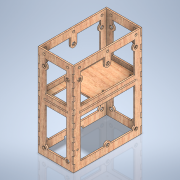
# Autodesk Inventor part: Skeleton
Saved by Autodesk Inventor 2020.2 (Build 242310000, 310)
## iProperties
Created: 2020-03-04
Part Number: Skeleton
Material: Wood (Birch)
Document SubType Name: Modeling
Designer: sdekr
Density: 0.55 g/cm^3
Appearance: Birch - Natural Polished
Author: sdekr
Autodesk Inventor part; units mm, degrees
sketch "Sketch1" plane through (0, 0, 0) normal (0, 1, 0) x (-1, 0, 0)
  line L0 (-37.5, 72.5) -> (37.5, 72.5)
  line L1 (37.5, 72.5) -> (37.5, -72.5)
  line L2 (37.5, -72.5) -> (-37.5, -72.5)
  line L3 (-37.5, -72.5) -> (-37.5, 72.5)
  line L4 (-37.5, 72.5) -> (37.5, -72.5) construction
  line L5 (37.5, 72.5) -> (-37.5, -72.5) construction
  point P0 (0, 0)
  dimension "d0" = 75
  dimension "d1" = 145
  constraints: 12 end point, 2 midpoint, 2 parallel, 1 horizontal, 1 perpendicular
  measures "d0" distance of L1.end L2.end
  measures "d1" distance of L0.end L1.end
surface extrude "ExtrusionSrf1" sketch "Sketch1" along normal blind 195 shown yes curves L0 L1 L2 L3
sketch "Sketch2" plane through (-37.5, 0, 72.5) normal (0, 0, 1) x (1, 0, 0)
  line L0 (0, 195) -> (75, 195) projected
  line L1 (75, 0) -> (75, 195) projected
  line L2 (0, 195) -> (75, 195)
  line L3 (75, 195) -> (75, 0)
  line L4 (75, 0) -> (0, 0)
  line L5 (0, 0) -> (0, 195)
  line L6 (15, 180) -> (60, 180)
  line L7 (60, 180) -> (60, 115)
  line L8 (60, 115) -> (15, 115)
  line L9 (15, 115) -> (15, 180)
  line L10 (15, 95) -> (60, 95)
  line L11 (60, 95) -> (60, 15)
  line L12 (60, 15) -> (15, 15)
  line L13 (15, 15) -> (15, 95)
  circle A0 centre (12.5, 187.5) radius 2.4
  circle A1 centre (62.5, 187.5) radius 2.4
  point P0 (37.5, 0)
  dimension "d4" = 15
  dimension "d5" = 15
  dimension "d6" = 15
  dimension "d7" = 15
  dimension "d8" = 15
  dimension "d9" = 20
  dimension "d12" = 4.8
  dimension "d13" = 4.8
  dimension "d14" = 7.5
  dimension "d15" = 7.5
  dimension "d16" = 12.5
  dimension "d17" = 12.5
  dimension "d81" = 80
  constraints: 24 end point, 6 parallel, 3 horizontal, 3 perpendicular, 2 centre point, 1 point on line
  measures "d4" distance between parallel lines of L1 L7
  measures "d5" distance between parallel lines of L5 L9
  measures "d6" distance between parallel lines of L4 L12
  measures "d7" distance between parallel lines of L0 L6
  measures "d8" distance between parallel lines of L5 L13
  measures "d9" distance between parallel lines of L10 L8
  measures "d12" diameter of A0
  measures "d13" diameter of A1
  measures "d14" distance from line of L0 A1.centre
  measures "d15" distance from line of L0 A0.centre
  measures "d16" distance from line of L5 A0.centre
  measures "d17" distance from line of L1 A1.centre
  measures "d81" distance of L10.end L11.end
extrude "Extrusion1" add sketch "Sketch2" against normal blind 3
ref_plane "Work Plane1" through (-37.5, 0, 0) normal (0, 0, 1) x (1, 0, 0)
sketch "Sketch5" plane through (-37.5, 0, 72.5) normal (0, 0, 1) x (1, 0, 0)
  line L0 (75, 0) -> (75, 195) projected
  line L1 (75, 180) -> (72, 180)
  line L2 (72, 180) -> (72, 165)
  line L3 (72, 165) -> (75, 165)
  line L4 (75, 165) -> (75, 180)
  line L5 (75, 195) -> (0, 195) projected
  line L6 (75, 155) -> (72, 155)
  line L7 (72, 155) -> (72, 140)
  line L8 (72, 140) -> (75, 140)
  line L9 (75, 140) -> (75, 155)
  line L10 (75, 130) -> (72, 130)
  line L11 (72, 130) -> (72, 115)
  line L12 (72, 115) -> (75, 115)
  line L13 (75, 115) -> (75, 130)
  line L14 (75, 105) -> (72, 105)
  line L15 (72, 105) -> (72, 90)
  line L16 (72, 90) -> (75, 90)
  line L17 (75, 90) -> (75, 105)
  line L18 (75, 80) -> (72, 80)
  line L19 (72, 80) -> (72, 65)
  line L20 (72, 65) -> (75, 65)
  line L21 (75, 65) -> (75, 80)
  line L22 (0, 0) -> (75, 0) projected
  line L23 (62.5, 106.5) -> (12.5, 106.5)
  line L24 (12.5, 106.5) -> (12.5, 103.5)
  line L25 (12.5, 103.5) -> (62.5, 103.5)
  line L26 (62.5, 103.5) -> (62.5, 106.5)
  line L27 (0, 195) -> (0, 0) projected
  line L28 (75, 55) -> (72, 55)
  line L29 (72, 55) -> (72, 40)
  line L30 (72, 40) -> (75, 40)
  line L31 (75, 40) -> (75, 55)
  line L32 (75, 30) -> (72, 30)
  line L33 (72, 30) -> (72, 15)
  line L34 (72, 15) -> (75, 15)
  line L35 (75, 15) -> (75, 30)
  line L36 (60, 115) -> (15, 115) projected
  line L37 (15, 95) -> (60, 95) projected
  point P0 (37.5, 0)
  point P1 (75, 90)
  point P2 (75, 65)
  point P3 (75, 115)
  point P4 (75, 140)
  point P5 (75, 165)
  point P6 (12.5, 105)
  point P7 (37.5, 103.5)
  point P8 (37.5, 195)
  dimension "d38" = 3
  dimension "d39" = 15
  dimension "d43" = 25
  dimension "d59" = 3
  dimension "d60" = 50
  dimension "d73" = 15
  dimension "d74" = 15
  dimension "d82" = 8.5
  dimension "d125" = 8.5
  constraints: 64 end point, 4 parallel, 3 midpoint, 2 horizontal, 2 perpendicular, 1 point on line, 1 vertical, 1 vertical alignment, 48 other
  measures "d38" distance of L1.start L1.end
  measures "d39" distance of L1.end L2.end
  measures "d43" distance of L1.start L6.start
  measures "d59" distance of L25.end L23.start
  measures "d60" distance of L23.start L23.end
  measures "d73" distance between parallel lines of L5 L1
  measures "d74" distance between parallel lines of L34 L22
  measures "d82" distance between parallel lines of L36 L23
  measures "d125" distance between parallel lines of L37 L25
extrude "Extrusion4" cut sketch "Sketch5" against normal up to surface (3 mm away) contours L34 L33 L32 L0 | L30 L29 L28 L0 | L0 L3 L2 L1 | L20 L19 L18 L0 | L0 L8 L7 L6 | L16 L15 L14 L0 | L0 L12 L11 L10 | L26 L25 L24 L23
ref_plane "Work Plane4" through (0, 195, 72.5) normal (1, 0, 0) x (0, 0, -1)
mirror "Mirror3" about plane through (0, 195, 72.5) normal (1, 0, 0) of "Extrusion4"
sketch "Sketch11" plane through (-37.5, 0, 69.5) normal (0, 0, -1) x (-1, 0, 0)
  circle A0 centre (-12.5, 165) radius 2.4 projected
  circle A1 centre (-62.5, 165) radius 2.4 projected
  circle A2 centre (-12.5, 15) radius 2.4 projected
  circle A3 centre (-62.5, 15) radius 2.4 projected
  line L0 (-60.6236, 168.25) -> (-58.7472, 165)
  line L1 (-58.7472, 165) -> (-60.6236, 161.75)
  line L2 (-60.6236, 161.75) -> (-64.3764, 161.75)
  line L3 (-64.3764, 161.75) -> (-66.2528, 165)
  line L4 (-66.2528, 165) -> (-64.3764, 168.25)
  line L5 (-64.3764, 168.25) -> (-60.6236, 168.25)
  line L6 (-14.3764, 168.25) -> (-10.6236, 168.25)
  line L7 (-10.6236, 168.25) -> (-8.7472, 165)
  line L8 (-8.7472, 165) -> (-10.6236, 161.75)
  line L9 (-10.6236, 161.75) -> (-14.3764, 161.75)
  line L10 (-14.3764, 161.75) -> (-16.2528, 165)
  line L11 (-16.2528, 165) -> (-14.3764, 168.25)
  line L12 (-10.6236, 18.25) -> (-8.7472, 15)
  line L13 (-8.7472, 15) -> (-10.6236, 11.75)
  line L14 (-10.6236, 11.75) -> (-14.3764, 11.75)
  line L15 (-14.3764, 11.75) -> (-16.2528, 15)
  line L16 (-16.2528, 15) -> (-14.3764, 18.25)
  line L17 (-14.3764, 18.25) -> (-10.6236, 18.25)
  line L18 (-60.6236, 18.25) -> (-58.7472, 15)
  line L19 (-58.7472, 15) -> (-60.6236, 11.75)
  line L20 (-60.6236, 11.75) -> (-64.3764, 11.75)
  line L21 (-64.3764, 11.75) -> (-66.2528, 15)
  line L22 (-66.2528, 15) -> (-64.3764, 18.25)
  line L23 (-64.3764, 18.25) -> (-60.6236, 18.25)
  circle A4 centre (-62.5, 165) radius 7
  circle A5 centre (-12.5, 165) radius 7
  circle A6 centre (-12.5, 15) radius 7
  circle A7 centre (-62.5, 15) radius 7
  point P0 (-37.5, 0)
  point P1 (-62.5, 18.25)
  dimension "d89" = 6.5
  dimension "d90" = 6.5
  dimension "d91" = 6.5
  dimension "d92" = 6.5
  dimension "d93" = 14
  dimension "d94" = 14
  dimension "d95" = 14
  dimension "d96" = 14
  constraints: 48 end point, 7 coincident, 4 centre point, 2 horizontal, 1 midpoint, 1 point on line, 52 other
  measures "d89" distance from line of point (-62.5, 18.25) L20
  measures "d90" distance between parallel lines of L14 L17
  measures "d91" distance between parallel lines of L2 L5
  measures "d92" distance between parallel lines of L9 L6
  measures "d93" diameter of A4
  measures "d94" diameter of A5
  measures "d95" diameter of A6
  measures "d96" diameter of A7
extrude "Extrusion10" add sketch "Sketch11" against normal up to surface (3 mm away) contours A4 | A5 | A6 | A7
extrude "Extrusion11" cut sketch "Sketch11" against normal through all contours A0 | A1 | A2 | A3 | L0 L1 L2 L3 L4 L5 | L6 L7 L8 L9 L10 L11 | L12 L13 L14 L15 L16 L17 | L18 L19 L20 L21 L22 L23
mirror "Mirror1" about plane through (-37.5, 0, 0) normal (0, 0, 1) of "Extrusion1", "Extrusion4", "Mirror3", "Extrusion10", "Extrusion11"
sketch "Sketch3" plane through (37.5, 0, 72.5) normal (1, 0, 0) x (0, 0, -1)
  line L0 (0, 195) -> (3, 195) projected
  line L1 (145, 0) -> (145, 195) projected
  line L2 (0, 195) -> (145, 195)
  line L3 (145, 195) -> (145, 0)
  line L4 (145, 0) -> (0, 0)
  line L5 (0, 0) -> (0, 195)
  line L6 (15, 180) -> (130, 180)
  line L7 (130, 180) -> (130, 115)
  line L8 (130, 115) -> (15, 115)
  line L9 (15, 115) -> (15, 180)
  line L10 (15, 96) -> (130, 96)
  line L11 (130, 96) -> (130, 15)
  line L12 (130, 15) -> (15, 15)
  line L13 (15, 15) -> (15, 96)
  circle A0 centre (12.5, 187.5) radius 2.4
  circle A1 centre (72.5, 187.5) radius 2.4
  circle A2 centre (132.5, 187.5) radius 2.4
  line L14 (12.5, 106.5) -> (132.5, 106.5)
  line L15 (132.5, 106.5) -> (132.5, 103.5)
  line L16 (132.5, 103.5) -> (12.5, 103.5)
  line L17 (12.5, 103.5) -> (12.5, 106.5)
  line L18 (145, 0) -> (145, 195) projected
  point P0 (72.5, 0)
  point P1 (145, 97.5)
  point P2 (72.5, 106.5)
  point P3 (72.5, 195)
  point P4 (0, 103.5)
  dimension "d18" = 15
  dimension "d19" = 15
  dimension "d20" = 15
  dimension "d21" = 15
  dimension "d23" = 4.8
  dimension "d24" = 4.8
  dimension "d25" = 4.8
  dimension "d26" = 12.5
  dimension "d27" = 7.5
  dimension "d28" = 7.5
  dimension "d29" = 7.5
  dimension "d30" = 12.5
  dimension "d61" = 3
  dimension "d62" = 120
  dimension "d83" = 8.5
  dimension "d126" = 81
  constraints: 32 end point, 8 parallel, 4 horizontal, 4 perpendicular, 3 centre point, 3 midpoint, 1 horizontal alignment, 1 point on line, 1 vertical alignment
  measures "d18" distance between parallel lines of L1 L7
  measures "d19" distance between parallel lines of L5 L9
  measures "d20" distance between parallel lines of L2 L6
  measures "d21" distance between parallel lines of L4 L12
  measures "d23" diameter of A0
  measures "d24" diameter of A1
  measures "d25" diameter of A2
  measures "d26" distance from line of L5 A0.centre
  measures "d27" distance from line of L2 A0.centre
  measures "d28" distance from line of L2 A1.centre
  measures "d29" distance from line of L2 A2.centre
  measures "d30" distance from line of L1 A2.centre
  measures "d61" distance of L14.end L15.end
  measures "d62" distance of L14.start L14.end
  measures "d83" distance between parallel lines of L8 L14
  measures "d126" distance of L10.end L11.end
extrude "Extrusion2" add sketch "Sketch3" against normal blind 3 separate body
sketch "Sketch12" plane through (34.5, 0, 72.5) normal (-1, 0, 0) x (0, 0, 1)
  circle A0 centre (-72.5, 165) radius 2.4 projected
  circle A1 centre (-132.5, 165) radius 2.4 projected
  circle A2 centre (-12.5, 165) radius 2.4 projected
  circle A3 centre (-72.5, 15) radius 2.4 projected
  circle A4 centre (-132.5, 15) radius 2.4 projected
  point P0 (-72.5, 0)
sketch "Sketch13" plane through (34.5, 0, 72.5) normal (-1, 0, 0) x (0, 0, 1)
  line L0 (-15, 15) -> (-130, 15) projected
  line L1 (-70.6236, 18.25) -> (-68.7472, 15)
  line L2 (-68.7472, 15) -> (-70.6236, 11.75)
  line L3 (-70.6236, 11.75) -> (-74.3764, 11.75)
  line L4 (-74.3764, 11.75) -> (-76.2528, 15)
  line L5 (-76.2528, 15) -> (-74.3764, 18.25)
  line L6 (-74.3764, 18.25) -> (-70.6236, 18.25)
  line L7 (-134.3764, 11.75) -> (-136.2528, 15)
  line L8 (-136.2528, 15) -> (-134.3764, 18.25)
  line L9 (-134.3764, 18.25) -> (-130.6236, 18.25)
  line L10 (-130.6236, 18.25) -> (-128.7472, 15)
  line L11 (-128.7472, 15) -> (-130.6236, 11.75)
  line L12 (-130.6236, 11.75) -> (-134.3764, 11.75)
  line L13 (-70.6236, 168.25) -> (-68.7472, 165)
  line L14 (-68.7472, 165) -> (-70.6236, 161.75)
  line L15 (-70.6236, 161.75) -> (-74.3764, 161.75)
  line L16 (-74.3764, 161.75) -> (-76.2528, 165)
  line L17 (-76.2528, 165) -> (-74.3764, 168.25)
  line L18 (-74.3764, 168.25) -> (-70.6236, 168.25)
  line L19 (-10.6236, 168.25) -> (-8.7472, 165)
  line L20 (-8.7472, 165) -> (-10.6236, 161.75)
  line L21 (-10.6236, 161.75) -> (-14.3764, 161.75)
  line L22 (-14.3764, 161.75) -> (-16.2528, 165)
  line L23 (-16.2528, 165) -> (-14.3764, 168.25)
  line L24 (-14.3764, 168.25) -> (-10.6236, 168.25)
  line L25 (-130.5927, 168.25) -> (-128.7163, 165)
  line L26 (-128.7163, 165) -> (-130.5927, 161.75)
  line L27 (-130.5927, 161.75) -> (-134.3455, 161.75)
  line L28 (-134.3455, 161.75) -> (-136.2219, 165)
  line L29 (-136.2219, 165) -> (-134.3455, 168.25)
  line L30 (-134.3455, 168.25) -> (-130.5927, 168.25)
  circle A0 centre (-132.5, 15) radius 7
  circle A1 centre (-72.5, 15) radius 7
  circle A2 centre (-12.5, 165) radius 7
  circle A3 centre (-132.4691, 165) radius 7
  circle A4 centre (-72.5, 165) radius 7
  line L31 (-79.5, 165) -> (-79.5, 180)
  line L32 (-130, 180) -> (-15, 180) projected
  line L33 (-65.5, 165) -> (-65.5, 180)
  point P0 (-72.5, 0)
  point P1 (-132.5, 15)
  point P2 (-132.5, 11.75)
  point P3 (-132.5, 15)
  point P4 (-65.5, 15)
  point P5 (-79.5, 15)
  dimension "d101" = 6.5
  dimension "d102" = 6.5
  dimension "d103" = 6.5
  dimension "d104" = 6.5
  dimension "d105" = 6.5
  dimension "d106" = 14
  dimension "d107" = 14
  dimension "d108" = 14
  dimension "d109" = 14
  dimension "d110" = 14
  constraints: 64 end point, 7 coincident, 5 centre point, 3 point on line, 2 horizontal, 2 midpoint, 2 point on circle, 2 vertical, 1 tangent, 65 other
  measures "d101" distance between parallel lines of L27 L30
  measures "d102" distance between parallel lines of L18 L15
  measures "d103" distance between parallel lines of L21 L24
  measures "d104" distance between parallel lines of L3 L6
  measures "d105" distance between parallel lines of L9 L12
  measures "d106" diameter of A0
  measures "d107" diameter of A1
  measures "d108" diameter of A2
  measures "d109" diameter of A3
  measures "d110" diameter of A4
extrude "Extrusion12" add sketch "Sketch13" against normal up to surface (3 mm away) contours L0 L1 L6 L5 A1 | A0 | A2 | A3 | A4 | A4 L31 L32 L33 bodies 2
extrude "Extrusion13" cut sketch "Sketch13" against normal up to surface (3 mm away) contours L2 L3 L4 L0 | L7 L8 L9 L10 L11 L12 | L19 L20 L21 L22 L23 L24 | L25 L26 L27 L28 L29 L30 bodies 2
sketch "Sketch6" plane through (37.5, 0, 72.5) normal (1, 0, 0) x (0, 0, -1)
  line L0 (0, 180) -> (3, 180) projected
  line L1 (3, 195) -> (3, 180) projected
  line L2 (0, 195) -> (3, 195) projected
  line L3 (0, 180) -> (0, 195) projected
  line L4 (3, 165) -> (0, 165) projected
  line L5 (0, 155) -> (0, 165) projected
  line L6 (0, 155) -> (3, 155) projected
  line L7 (3, 165) -> (3, 155) projected
  line L8 (0, 130) -> (3, 130) projected
  line L9 (3, 140) -> (3, 130) projected
  line L10 (3, 140) -> (0, 140) projected
  line L11 (0, 130) -> (0, 140) projected
  line L12 (3, 115) -> (0, 115) projected
  line L13 (0, 105) -> (0, 115) projected
  line L14 (0, 105) -> (3, 105) projected
  line L15 (3, 115) -> (3, 105) projected
  line L16 (3, 90) -> (0, 90) projected
  line L17 (0, 80) -> (0, 90) projected
  line L18 (0, 80) -> (3, 80) projected
  line L19 (3, 90) -> (3, 80) projected
  line L20 (3, 65) -> (0, 65) projected
  line L21 (0, 0) -> (0, 15) projected
  line L22 (0, 0) -> (3, 0) projected
  line L23 (3, 15) -> (3, 0) projected
  line L24 (0, 30) -> (3, 30) projected
  line L25 (3, 40) -> (3, 30) projected
  line L26 (3, 40) -> (0, 40) projected
  line L27 (0, 30) -> (0, 40) projected
  line L28 (3, 15) -> (0, 15) projected
  line L29 (0, 180) -> (3, 180) projected
  line L30 (3, 195) -> (3, 180) projected
  line L31 (0, 195) -> (3, 195) projected
  line L32 (0, 180) -> (0, 195) projected
  line L33 (3, 165) -> (0, 165) projected
  line L34 (0, 155) -> (0, 165) projected
  line L35 (0, 155) -> (3, 155) projected
  line L36 (3, 165) -> (3, 155) projected
  line L37 (3, 140) -> (0, 140) projected
  line L38 (0, 130) -> (0, 140) projected
  line L39 (0, 130) -> (3, 130) projected
  line L40 (3, 140) -> (3, 130) projected
  line L41 (0, 105) -> (3, 105) projected
  line L42 (3, 115) -> (3, 105) projected
  line L43 (3, 115) -> (0, 115) projected
  line L44 (0, 105) -> (0, 115) projected
  line L45 (0, 55) -> (3, 55) projected
  line L46 (3, 65) -> (3, 55) projected
  line L47 (0, 55) -> (0, 65) projected
  line L48 (3, 90) -> (0, 90) projected
  line L49 (0, 80) -> (0, 90) projected
  line L50 (0, 80) -> (3, 80) projected
  line L51 (3, 90) -> (3, 80) projected
  point P0 (72.5, 0)
extrude "Extrusion5" cut sketch "Sketch6" against normal up to surface (3 mm away) bodies 2
ref_plane "Work Plane2" through (0, 0, 72.5) normal (1, 0, 0) x (0, 0, -1)
mirror "Mirror5" about plane through (-37.5, 0, 0) normal (0, 0, 1) of "Extrusion5" bodies 2
mirror "Mirror4" about plane through (0, 0, 72.5) normal (1, 0, 0) bodies 2
ref_plane "Work Plane5" through (-37.5, 105, 72.5) normal (0, 1, 0) x (1, 0, 0)
sketch "Sketch8" plane through (-37.5, 105, 72.5) normal (0, 1, 0) x (1, 0, 0)
  line L0 (12.5, 0) -> (12.5, 3) projected
  line L1 (0, 12.5) -> (3, 12.5) projected
  line L2 (75, 12.5) -> (72, 12.5) projected
  line L3 (62.5, 0) -> (62.5, 3) projected
  line L4 (62.5, 145) -> (62.5, 142) projected
  line L5 (12.5, 145) -> (12.5, 142) projected
  line L6 (75, 132.5) -> (72, 132.5) projected
  line L7 (0, 132.5) -> (3, 132.5) projected
  line L8 (0, 12.5) -> (0, 132.5)
  line L9 (3, 132.5) -> (3, 142)
  line L10 (3, 142) -> (12.5, 142)
  line L11 (12.5, 145) -> (62.5, 145)
  line L12 (72, 132.5) -> (72, 142)
  line L13 (72, 142) -> (62.5, 142)
  line L14 (75, 132.5) -> (75, 12.5)
  line L15 (72, 12.5) -> (72, 3)
  line L16 (72, 3) -> (62.5, 3)
  line L17 (62.5, 0) -> (12.5, 0)
  line L18 (12.5, 3) -> (3, 3)
  line L19 (3, 3) -> (3, 12.5)
  line L20 (15, 15) -> (60, 15)
  line L21 (60, 15) -> (60, 50)
  line L22 (60, 50) -> (15, 50)
  line L23 (15, 50) -> (15, 15)
  point P0 (37.5, 72.5)
  dimension "d75" = 15
  dimension "d76" = 15
  dimension "d77" = 15
  dimension "d78" = 35
  constraints: 32 end point, 7 perpendicular, 3 parallel, 3 vertical, 2 point on line, 1 horizontal
  measures "d75" distance between parallel lines of L8 L23
  measures "d76" distance between parallel lines of L17 L20
  measures "d77" distance between parallel lines of L14 L21
  measures "d78" distance of L22.end L20.start
extrude "Extrusion7" add sketch "Sketch8" along normal mid plane 3 separate body
sketch "Sketch9" plane through (37.5, 0, 72.5) normal (1, 0, 0) x (0, 0, -1)
  circle A0 centre (8.5, 38.45) radius 1.75 projected
  point P0 (72.5, 0)
extrude "Extrusion8" cut sketch "Sketch9" against normal through all bodies 2
sketch "Sketch10" plane through (-37.5, 165, -72.5) normal (-1, 0, 0) x (0, 0, 1)
  line L0 (52.5, -160) -> (92.5, -160) projected
  line L1 (92.5, -160) -> (92.5, -165) projected
  line L2 (52.5, -165) -> (52.5, -160) projected
  line L3 (52.5, -165) -> (92.5, -165)
  line L4 (3, -165) -> (142, -165) projected
  point P0 (72.5, -165)
  constraints: 2 end point, 1 collinear
extrude "Extrusion9" cut sketch "Sketch10" against normal blind 5 bodies 2
sketch "Sketch14" plane through (-37.5, 15, 72.5) normal (-1, 0, 0) x (0, 0, 1)
  line L0 (-130.6236, 3.25) -> (-134.3764, 3.25) projected
  line L1 (-128.7472, 0) -> (-130.6236, 3.25) projected
  line L2 (-130.6236, -3.25) -> (-128.7472, 0) projected
  line L3 (-134.3764, -3.25) -> (-130.6236, -3.25) projected
  line L4 (-136.2528, 0) -> (-134.3764, -3.25) projected
  line L5 (-134.3764, 3.25) -> (-136.2528, 0) projected
  arc A0 (-125.5, 0) -> (-130, 6.5383) centre (-132.5, 0) ccw projected
  line L6 (-72.5, -15) -> (-72.5, 20.3561)
  line L7 (-14.3764, 3.25) -> (-10.6236, 3.25)
  line L8 (-16.2528, 0) -> (-14.3764, 3.25)
  line L9 (-14.3764, -3.25) -> (-16.2528, 0)
  line L10 (-10.6236, -3.25) -> (-14.3764, -3.25)
  line L11 (-8.7472, 0) -> (-10.6236, -3.25)
  line L12 (-10.6236, 3.25) -> (-8.7472, 0)
  arc A1 (-15, 6.5383) -> (-19.5, 0) centre (-12.5, 0) ccw
  circle A2 centre (-12.5, 0) radius 7
  constraints: 14 end point, 9 symmetric about line, 2 centre point, 2 point on circle, 1 coincident, 1 concentric, 1 vertical, 1 other
extrude "Extrusion14" add sketch "Sketch14" against normal up to surface (3 mm away) contours A2 A1 bodies 2
extrude "Extrusion15" cut sketch "Sketch14" against normal up to surface (3 mm away) contours L7 L12 L11 L10 L9 L8 bodies 2
sketch "Sketch15" plane through (-37.5, 106.5, 72.5) normal (0, 1, 0) x (1, 0, 0)
  circle A0 centre (62, 75.5) radius 1.375 projected
  circle A1 centre (13, 75.5) radius 1.375 projected
  circle A2 centre (62, 133.5) radius 1.375 projected
  circle A3 centre (13, 133.5) radius 3 projected
  circle A4 centre (62, 133.5) radius 1.5
  circle A5 centre (13, 133.5) radius 1.5
  circle A6 centre (62, 75.5) radius 1.5
  circle A7 centre (13, 75.5) radius 1.5
  point P0 (37.5, 72.5)
  dimension "d119" = 3
  dimension "d120" = 3
  dimension "d121" = 3
  dimension "d122" = 3
  constraints: 4 centre point, 4 coincident
  measures "d119" diameter of A4
  measures "d120" diameter of A5
  measures "d121" diameter of A6
  measures "d122" diameter of A7
extrude "Extrusion16" cut sketch "Sketch15" against normal up to surface (3 mm away) contours A0 | A1 | A2 | A4 | A5 | A6 | A7 bodies 3
equation "\"d15\" = d14"
equation "\"d16\" = d17"
equation "\"d26\" = d30"
body "Solid1"
body "Srf1"
body "Solid2"
body "Solid4"
